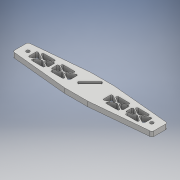
# Autodesk Inventor part: gyromount
Saved by Autodesk Inventor 2018.3 (Build 223284000, 284)
## iProperties
Created: 2018-12-20
Part Number: gyromount
Material: 一般
Document SubType Name: Modeling
Designer: shun2
Density: 1 g/cm^3
Appearance: 既定
Author: shun2
Autodesk Inventor part; units mm, degrees
ref_plane "YZ Plane" through (0, 0, 0) normal (1, 0, 0) x (0, 1, 0)
ref_plane "XZ Plane" through (0, 0, 0) normal (0, 1, 0) x (-1, 0, 0)
ref_plane "XY Plane" through (0, 0, 0) normal (0, 0, 1) x (1, 0, 0)
sketch "スケッチ1" plane through (0, 0, 0) normal (0, 0, 1) x (1, 0, 0)
  circle A0 centre (0, 0) radius 1.7
  circle A1 centre (126.625, 0) radius 1.7
  line L0 (134.804, -5.9762) -> (134.804, 6.0238)
  line L1 (-7.821, 6.0238) -> (-7.821, -5.9762)
  arc A2 (-5.821, 8.0238) -> (-7.821, 6.0238) centre (-5.821, 6.0238) ccw
  arc A3 (-7.821, -5.9762) -> (-5.821, -7.9762) centre (-5.821, -5.9762) ccw
  arc A4 (134.804, 6.0238) -> (132.804, 8.0238) centre (132.804, 6.0238) ccw
  arc A5 (132.804, -7.9762) -> (134.804, -5.9762) centre (132.804, -5.9762) ccw
  line L2 (63.4551, -0.0131) -> (60.6266, 2.8153)
  line L3 (60.6266, 2.8153) -> (54.9698, -2.8415)
  line L4 (60.6266, 2.8153) -> (68.6266, 2.8153) construction
  line L5 (60.6266, 2.8153) -> (66.3034, 8.4921)
  line L6 (60.6266, 2.8153) -> (68.6548, 2.8153) construction
  line L7 (66.3232, 9.8858) -> (65.6371, 10.6123)
  line L8 (53.5556, -2.8414) -> (52.8485, -2.1343)
  line L9 (52.8486, -0.7201) -> (64.2031, 10.6328)
  line L10 (50.8558, 13.4563) -> (74.7634, 13.4563)
  arc A6 (52.8486, -0.7201) -> (52.8485, -2.1343) centre (53.5557, -1.4273) ccw
  arc A7 (53.5556, -2.8414) -> (54.9698, -2.8415) centre (54.2627, -2.1344) ccw
  arc A8 (65.6371, 10.6123) -> (64.2031, 10.6328) centre (64.9101, 9.9256) ccw
  arc A9 (66.3034, 8.4921) -> (66.3232, 9.8858) centre (65.5963, 9.1992) ccw
  arc A10 (15.9698, -0.7397) -> (14.7602, -0.7647) centre (15.3856, -1.7515) ccw
  line L11 (15.9698, -0.7397) -> (21.6953, -4.0454)
  arc A11 (21.1112, -6.2255) -> (21.6953, -4.0454) centre (21.1112, -5.0572) ccw
  line L12 (21.1112, -6.2255) -> (10.1699, -6.2255)
  arc A12 (9.5444, -4.0704) -> (10.1699, -6.2255) centre (10.1699, -5.0572) ccw
  line L13 (9.5444, -4.0704) -> (14.7602, -0.7647)
  arc A13 (22.6232, -3.4465) -> (24.325, -2.4071) centre (23.1567, -2.4071) ccw
  line L14 (22.6232, -3.4465) -> (17.9962, -1.0715)
  arc A14 (17.9949, 1.0066) -> (17.9962, -1.0715) centre (18.5297, -0.0321) ccw
  line L15 (17.9949, 1.0066) -> (22.6263, 3.3666)
  arc A15 (24.325, 2.3257) -> (22.6263, 3.3666) centre (23.1567, 2.3257) ccw
  line L16 (24.325, 2.3257) -> (24.325, -2.4071)
  arc A16 (10.1699, 6.1672) -> (9.5444, 4.0121) centre (10.1699, 4.9989) ccw
  line L17 (10.1699, 6.1672) -> (21.1112, 6.1672)
  arc A17 (21.6953, 3.9871) -> (21.1112, 6.1672) centre (21.1112, 4.9989) ccw
  line L18 (21.6953, 3.9871) -> (15.9698, 0.6815)
  arc A18 (14.7602, 0.7065) -> (15.9698, 0.6815) centre (15.3856, 1.6933) ccw
  line L19 (14.7602, 0.7065) -> (9.5444, 4.0121)
  arc A19 (6.3779, 4.3006) -> (4.6749, 3.2743) centre (5.8431, 3.2619) ccw
  line L20 (6.3779, 4.3006) -> (12.7763, 1.0066)
  arc A20 (12.775, -1.0715) -> (12.7763, 1.0066) centre (12.2415, -0.0321) ccw
  line L21 (12.775, -1.0715) -> (6.3064, -4.3918)
  arc A21 (4.6046, -3.34) -> (6.3064, -4.3918) centre (5.7729, -3.3524) ccw
  line L22 (4.6046, -3.34) -> (4.6749, 3.2743)
  arc A22 (30.2166, 6.1672) -> (29.6325, 3.9871) centre (30.2166, 4.9989) ccw
  arc A23 (28.7015, 3.3666) -> (27.0028, 2.3257) centre (28.1711, 2.3257) ccw
  arc A24 (29.6325, -4.0454) -> (30.2166, -6.2255) centre (30.2166, -5.0572) ccw
  arc A25 (27.0028, -2.4071) -> (28.7046, -3.4465) centre (28.1711, -2.4071) ccw
  line L23 (33.3328, 1.0066) -> (28.7015, 3.3666)
  arc A26 (33.3316, -1.0715) -> (33.3328, 1.0066) centre (32.7981, -0.0321) ccw
  line L24 (28.7046, -3.4465) -> (33.3316, -1.0715)
  line L25 (29.6325, 3.9871) -> (35.358, 0.6815)
  arc A27 (35.358, 0.6815) -> (36.5676, 0.7065) centre (35.9422, 1.6933) ccw
  arc A28 (36.5676, -0.7647) -> (35.358, -0.7397) centre (35.9422, -1.7515) ccw
  line L26 (35.358, -0.7397) -> (29.6325, -4.0454)
  line L27 (41.1579, 6.1672) -> (30.2166, 6.1672)
  line L28 (30.2166, -6.2255) -> (41.1579, -6.2255)
  line L29 (27.0028, 2.3257) -> (27.0028, -2.4071)
  arc A29 (38.5515, 1.0066) -> (38.5528, -1.0715) centre (39.0863, -0.0321) ccw
  line L30 (36.5676, 0.7065) -> (41.7834, 4.0121)
  line L31 (41.7834, -4.0704) -> (36.5676, -0.7647)
  arc A30 (41.7834, 4.0121) -> (41.1579, 6.1672) centre (41.1579, 4.9989) ccw
  arc A31 (41.1579, -6.2255) -> (41.7834, -4.0704) centre (41.1579, -5.0572) ccw
  line L32 (44.9499, 4.3006) -> (38.5515, 1.0066)
  line L33 (38.5528, -1.0715) -> (45.0214, -4.3918)
  line L34 (46.7232, -3.34) -> (46.6529, 3.2743)
  arc A32 (45.0214, -4.3918) -> (46.7232, -3.34) centre (45.5549, -3.3524) ccw
  arc A33 (46.6529, 3.2743) -> (44.9499, 4.3006) centre (45.4847, 3.2619) ccw
  arc A34 (97.9717, 3.9871) -> (97.3875, 6.1672) centre (97.3875, 4.9989) ccw
  arc A35 (100.6014, 2.3257) -> (98.9026, 3.3666) centre (99.4331, 2.3257) ccw
  arc A36 (97.3875, -6.2255) -> (97.9717, -4.0454) centre (97.3875, -5.0572) ccw
  arc A37 (98.8996, -3.4465) -> (100.6014, -2.4071) centre (99.4331, -2.4071) ccw
  line L35 (94.2713, 1.0066) -> (98.9026, 3.3666)
  arc A38 (94.2713, 1.0066) -> (94.2726, -1.0715) centre (94.8061, -0.0321) ccw
  line L36 (98.8996, -3.4465) -> (94.2726, -1.0715)
  line L37 (97.9717, 3.9871) -> (92.2461, 0.6815)
  arc A39 (91.0366, 0.7065) -> (92.2461, 0.6815) centre (91.662, 1.6933) ccw
  arc A40 (92.2461, -0.7397) -> (91.0366, -0.7647) centre (91.662, -1.7515) ccw
  line L38 (92.2461, -0.7397) -> (97.9717, -4.0454)
  line L39 (86.4462, 6.1672) -> (97.3875, 6.1672)
  line L40 (97.3875, -6.2255) -> (86.4462, -6.2255)
  line L41 (100.6014, 2.3257) -> (100.6014, -2.4071)
  arc A41 (89.0514, -1.0715) -> (89.0527, 1.0066) centre (88.5179, -0.0321) ccw
  line L42 (91.0366, 0.7065) -> (85.8208, 4.0121)
  line L43 (85.8208, -4.0704) -> (91.0366, -0.7647)
  arc A42 (86.4462, 6.1672) -> (85.8208, 4.0121) centre (86.4462, 4.9989) ccw
  arc A43 (85.8208, -4.0704) -> (86.4462, -6.2255) centre (86.4462, -5.0572) ccw
  line L44 (82.6542, 4.3006) -> (89.0527, 1.0066)
  line L45 (89.0514, -1.0715) -> (82.5827, -4.3918)
  line L46 (80.881, -3.34) -> (80.9512, 3.2743)
  arc A44 (80.881, -3.34) -> (82.5827, -4.3918) centre (82.0492, -3.3524) ccw
  arc A45 (82.6542, 4.3006) -> (80.9512, 3.2743) centre (82.1195, 3.2619) ccw
  arc A46 (111.6344, 0.6815) -> (112.8439, 0.7065) centre (112.2185, 1.6933) ccw
  arc A47 (112.8439, -0.7647) -> (111.6344, -0.7397) centre (112.2185, -1.7515) ccw
  line L47 (117.4343, 6.1672) -> (106.493, 6.1672)
  line L48 (106.493, -6.2255) -> (117.4343, -6.2255)
  line L49 (112.8439, 0.7065) -> (118.0597, 4.0121)
  line L50 (118.0597, -4.0704) -> (112.8439, -0.7647)
  arc A48 (117.4343, -6.2255) -> (118.0597, -4.0704) centre (117.4343, -5.0572) ccw
  arc A49 (114.8279, 1.0066) -> (114.8291, -1.0715) centre (115.3626, -0.0321) ccw
  arc A50 (109.6079, -1.0715) -> (109.6092, 1.0066) centre (109.0744, -0.0321) ccw
  line L51 (105.9088, 3.9871) -> (111.6344, 0.6815)
  line L52 (109.6092, 1.0066) -> (104.9779, 3.3666)
  line L53 (111.6344, -0.7397) -> (105.9088, -4.0454)
  line L54 (104.981, -3.4465) -> (109.6079, -1.0715)
  arc A51 (106.493, 6.1672) -> (105.9088, 3.9871) centre (106.493, 4.9989) ccw
  arc A52 (104.9779, 3.3666) -> (103.2791, 2.3257) centre (104.4475, 2.3257) ccw
  line L55 (103.2791, 2.3257) -> (103.2791, -2.4071)
  arc A53 (103.2791, -2.4071) -> (104.981, -3.4465) centre (104.4475, -2.4071) ccw
  arc A54 (105.9088, -4.0454) -> (106.493, -6.2255) centre (106.493, -5.0572) ccw
  line L56 (121.2263, 4.3006) -> (114.8279, 1.0066)
  line L57 (114.8291, -1.0715) -> (121.2978, -4.3918)
  arc A55 (122.9293, 3.2743) -> (121.2263, 4.3006) centre (121.761, 3.2619) ccw
  line L58 (122.9995, -3.34) -> (122.9293, 3.2743)
  arc A56 (121.2978, -4.3918) -> (122.9995, -3.34) centre (121.8313, -3.3524) ccw
  arc A57 (118.0597, 4.0121) -> (117.4343, 6.1672) centre (117.4343, 4.9989) ccw
  line L59 (-5.821, 8.0238) -> (50.8558, 13.4563)
  line L60 (74.7634, 13.4563) -> (132.9901, 8.0151)
  line L61 (50.8558, -13.5217) -> (74.7634, -13.5217)
  line L62 (74.7634, -13.5217) -> (132.804, -7.9762)
  line L63 (-5.821, -7.9762) -> (50.8558, -13.5217)
  point P0 (134.804, 8.0238)
  point P1 (134.804, -7.9762)
  point P2 (-7.821, 8.0238)
  point P3 (54.2627, -3.5487)
  point P4 (66.9906, 9.1793)
  point P5 (64.9306, 11.3602)
  point P6 (52.1415, -1.4272)
  point P7 (15.0236, -1.4895)
  point P8 (36.3042, -1.4895)
  point P9 (91.3, -1.4895)
  point P10 (112.5805, -1.4895)
  dimension "d0" = 3.4
  dimension "d1" = 3.4
  dimension "d3" = 142.625
  dimension "d4" = 16
  dimension "d5" = 2
  dimension "d6" = 2
  dimension "d19" = 4
  dimension "d22" = 9
  dimension "d23" = 135
  dimension "d24" = 9
  dimension "d25" = 45
  dimension "d29" = 3
  dimension "d30" = 3
  dimension "d33" = 1
  constraints: 128 end point, 113 point on circle, 58 centre point, 13 tangent, 11 point on line, 5 equal radius, 4 horizontal, 2 equal length, 1 coincident, 1 collinear, 1 parallel, 1 perpendicular
  measures "d0" diameter of A0
  measures "d1" diameter of A1
  measures "d3" distance of point (-7.821, 8.024) point (134.804, 8.024)
  measures "d4" distance of point (134.804, 8.024) point (134.804, -7.976)
  measures "d5" radius of A2
  measures "d6" radius of A3
  measures "d19" distance of L2.start L2.end
  measures "d22" distance of L2.end point (54.263, -3.549)
  measures "d23" angle of L3 L4
  measures "d24" distance of L2.end point (66.991, 9.179)
  measures "d25" angle of L6 L5
  measures "d29" distance of point (66.991, 9.179) point (64.931, 11.36)
  measures "d30" distance of point (54.263, -3.549) point (52.141, -1.427)
  measures "d33" radius of A6
extrude "押し出し1" add sketch "スケッチ1" along normal blind 5
